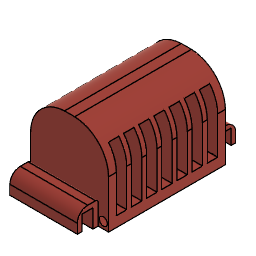
Tensor acoplable (Autodesk Fusion 360 design; units mm, degrees)
Autodesk Fusion 360 part; units mm, degrees
note: some values were not read from the file. Chosen so that the rebuilt part matches the saved one: which pieces of a blend or face edit are solid. Set by a fixed rule: which sketch regions a step uses.
sketch "Boceto1" plane through (0, 0, 0) normal (1, 0, 0) x (0, 1, 0)
  line L0 (0, 0) -> (0, 5)
  line L1 (0, 5) -> (4, 5)
  line L2 (4, 5) -> (4, 0)
  line L3 (4, 0) -> (53, 0)
  line L4 (53, 0) -> (53, 5)
  line L5 (53, 5) -> (57, 5)
  line L6 (57, 5) -> (57, 0)
  line L7 (-2, 0) -> (-2, 7)
  line L8 (-2, 7) -> (6, 7)
  line L9 (6, 7) -> (6, 2)
  line L10 (6, 2) -> (51, 2)
  line L11 (51, 2) -> (51, 7)
  line L12 (51, 7) -> (59, 7)
  line L13 (59, 7) -> (59, 0)
  line L14 (-2, 0) -> (0, 0)
  line L15 (59, 0) -> (57, 0)
  dimension "d1" = 5
  dimension "d2" = 4
  dimension "d3" = 49
  dimension "d4" = 5
  dimension "d5" = 4
  dimension "d6" = 5
  dimension "d7" = -2
  constraint coincident L0.start L14.end
  constraint vertical L0
  constraint perpendicular L0 L1
  constraint perpendicular L1 L2
  constraint perpendicular L2 L3
  constraint perpendicular L3 L4
  constraint perpendicular L4 L5
  constraint perpendicular L5 L6
  constraint perpendicular L0 L14
  constraint perpendicular L13 L15
  measures "d1" distance of L0.start L0.end
  measures "d2" distance of L0.end L1.end
  measures "d3" distance of L2.end L3.end
  measures "d4" distance of L3.end L4.end
  measures "d5" distance of L4.end L5.end
  measures "d6" distance of L5.end L6.end
extrude "Extruir1" add sketch "Boceto1" along normal blind 30 makes body 1
extrude "Extruir3" cut 1 faces at (10, 21, 2) along direction (0, 0, -1) blind 0.5 on bodies 1 bodies 1
sketch "Boceto2" plane through (0, 51, 0) normal (0, -1, 0) x (1, 0, 0)
  line L0 (0, 7) -> (0, 1.5)
  line L1 (30, 1.5) -> (30, 7)
  line L2 (30, 7) -> (0, 7)
  line L3 (0, 1.5) -> (30, 1.5)
  line L4 (15, 1.5) -> (15, 5)
  arc A0 (30, 1.5) -> (0, 1.5) centre (15, -28.8929) ccw
  dimension "d15" = 3.5
  constraint midpoint L3 L4.start
  constraint perpendicular L3 L4
  constraint coincident L4.end A0
  constraint coincident L1.start L3.end
  constraint coincident L0.end L3.start
  measures "d15" distance of L4.start L4.end
extrude "Extruir2" add sketch "Boceto2" along normal up to surface (45 mm away) contours L3 L4 A0 | L3 L4 A0 bodies 1
copy_body "Cuerpo - > Comp.1" bodies 1 removing the originals makes body 2 in component "Rodillo acoplable"
move_face "CarasDesfase1" offset -0.2 2 faces at (10, 57, 3.3333) (10, 0, 1.6667) on bodies 2 in component "Rodillo acoplable"
fillet "Empalme1" radius 4 2 edges at (15, -2, 7) (15, 59, 7) on bodies 2 in component "Rodillo acoplable"
fillet "Empalme2" radius 1 2 edges at (15, 6, 7) (15, 51, 7) on bodies 2 in component "Rodillo acoplable"
move_face "CarasDesfase2" offset 25 1 faces at (1.3409, 21, 2.1258) on bodies 2 in component "Rodillo acoplable"
fillet "Empalme3" radius 13.5 2 edges at (30, 28.5, 28.0577) (0, 28.5, 28.0577) on bodies 2 in component "Rodillo acoplable"
extrude "Extruir1'" add 2 faces at (10, -1.4, 0) (10, 58.4, 0) along direction (0, 0, -1) blind 1 on bodies 2 bodies 2 in component "Rodillo acoplable"
sketch "Boceto3" plane through (0, -0.2, 0) normal (0, 1, 0) x (-1, 0, 0)
  line L0 (0, -1) -> (0, 5)
  line L1 (0, 5) -> (-30, 5)
  line L2 (-30, 5) -> (-30, -1)
  line L3 (-30, -1) -> (0, -1)
  line L4 (0, -1) -> (-30, -1)
  line L5 (-30, -1) -> (-30, 1.5)
  line L6 (-30, 1.5) -> (0, 1.5)
  line L7 (0, 1.5) -> (0, -1)
  dimension "d38" = 2.5
  constraint horizontal L4
  constraint vertical L5
  constraint horizontal L6
  constraint vertical L7
  constraint coincident L2 L5.end
  constraint coincident L0.start L3.end
  measures "d38" distance of L2.end L5.end
extrude "Extruir9" add sketch "Boceto3" along normal blind 1.25 contours L0 L2 L3 L4 L5 L6 L7 bodies 2 in component "Rodillo acoplable"
sketch "Boceto4" plane through (0, 57.2, 0) normal (0, -1, 0) x (1, 0, 0)
  line L0 (0, 5) -> (0, -1)
  line L1 (0, -1) -> (30, -1)
  line L2 (30, -1) -> (30, 5)
  line L3 (30, 5) -> (0, 5)
  line L4 (0, -1) -> (30, -1)
  line L5 (30, -1) -> (30, 1.5)
  line L6 (30, 1.5) -> (0, 1.5)
  line L7 (0, 1.5) -> (0, -1)
  dimension "d27" = 2.5
  constraint horizontal L4
  constraint vertical L5
  constraint horizontal L6
  constraint vertical L7
  constraint coincident L0.end L1.start
  measures "d27" distance of L0.end L6.end
extrude "Extruir3'" add sketch "Boceto4" along normal blind 1.25 contours L0 L1 L2 L4 L5 L6 L7 bodies 2 in component "Rodillo acoplable"
extrude "Extruir4" add 1 faces at (20, 36.6667, 0) along direction (0, 0, -1) blind 1 on bodies 2 bodies 2 in component "Rodillo acoplable"
sketch "Boceto5" plane through (30, 0, 0) normal (1, 0, 0) x (0, 1, 0)
  line L0 (51, 16.4752) -> (6, 16.4752)
  line L1 (6, 16.4752) -> (6, 6)
  arc A0 (6, 6) -> (5, 7) centre (5, 6) ccw
  line L2 (5, 7) -> (2, 7)
  arc A1 (2, 7) -> (-2, 3) centre (2, 3) ccw
  line L3 (-2, 3) -> (-2, -1)
  line L4 (-2, -1) -> (-0.2, -1)
  line L5 (-0.2, 1.5) -> (-0.2, 5)
  line L6 (-0.2, 5) -> (4, 5)
  line L7 (4, 5) -> (4, -1)
  line L8 (4, -1) -> (53, -1)
  line L9 (53, -1) -> (53, 5)
  line L10 (53, 5) -> (57.2, 5)
  line L11 (57.2, 5) -> (57.2, 1.5)
  line L12 (57.2, 1.5) -> (55.95, 1.5)
  line L13 (55.95, 1.5) -> (55.95, -1)
  line L14 (55.95, -1) -> (59, -1)
  line L15 (59, -1) -> (59, 3)
  arc A2 (59, 3) -> (55, 7) centre (55, 3) ccw
  line L16 (55, 7) -> (52, 7)
  arc A3 (52, 7) -> (51, 6) centre (52, 6) ccw
  line L17 (51, 6) -> (51, 16.4752)
  line L18 (6, 6) -> (6, -1)
  line L19 (51, 6) -> (51, -1)
  line L20 (-0.2, -1) -> (-0.2, 1.5)
  constraint coincident L1.end A0.start
  constraint coincident L8 L18.end
  constraint tangent A0 L18
  constraint coincident A3.end L17.start
  constraint coincident L8 L19.end
  constraint tangent A3 L19
extrude "Extruir5" cut sketch "Boceto5" against normal blind 4 contours L8 L9 L10 L11 L12 L13 L14 L15 A2 L16 A3 L19 | A0 L2 A1 L3 L4 L5 L6 L7 L8 L18 L20 bodies 2 in component "Rodillo acoplable"
sketch "Boceto7" plane through (0, 51, 0) normal (0, 1, 0) x (-1, 0, 0)
  arc A0 (0, 16.4752) -> (-13.0539, 29.9678) centre (-13.5, 16.4752) ccw
  arc A1 (-13.0539, 29.9678) -> (-16.9461, 29.9678) centre (-15, -28.8929) ccw
  arc A2 (-16.9461, 29.9678) -> (-30, 16.4752) centre (-16.5, 16.4752) ccw
  line L0 (-30, 16.4752) -> (-30, -1)
  line L1 (-30, -1) -> (-26, -1)
  line L2 (-26, -1) -> (-26, 6)
  line L3 (-26, 6) -> (0, 6)
  line L4 (0, 6) -> (0, 16.4752)
  line L5 (-28, -1) -> (-28, 0.6)
  circle A3 centre (-28, 0.6) radius 1.55
  dimension "d41" = 1.6
  dimension "d42" = 3.1
  constraint midpoint L1 L5.start
  constraint perpendicular L1 L5
  constraint coincident L5.end A3.centre
  measures "d41" distance of L5.start L5.end
  measures "d42" diameter of A3
extrude "Extruir8" cut sketch "Boceto7" against normal blind 45 contours A3 bodies 2 in component "Rodillo acoplable"
extrude "Extruir10" cut 1 faces at (30, 0.2167, -0.1667) along direction (-1, 0, 0) up to surface (4 mm away) on bodies 2 bodies 2 in component "Rodillo acoplable"
extrude "Extruir11" add sketch "Boceto7" against normal blind 42 contours A3 bodies 2 in component "Rodillo acoplable"
extrude "Extruir12" cut sketch "Boceto7" against normal blind 3 contours A3 bodies 2 in component "Rodillo acoplable"
extrude "Extruir13" cut 2 faces at (17.3333, 2.6, 5) (8.6667, 54.4, 5) along direction (0, 0, 1) blind 0.15 on bodies 2 bodies 2 in component "Rodillo acoplable"
sketch "Boceto8" plane through (30, 0, 0) normal (1, 0, 0) x (0, 1, 0)
  line L0 (6, 16.4752) -> (6, -1)
  line L1 (6, -1) -> (51, -1)
  line L2 (51, -1) -> (51, 16.4752)
  line L3 (51, 16.4752) -> (6, 16.4752)
  line L4 (6, -1) -> (9, -1)
  line L5 (9, -1) -> (9, 2)
  line L6 (9, 2) -> (13, 2)
  line L7 (13, 2) -> (13, 25)
  line L8 (13, 25) -> (9, 25)
  line L9 (9, 25) -> (9, 2)
  line L10 (18.8333, 2) -> (18.8333, 25)
  line L11 (18.8333, 25) -> (14.8333, 25)
  line L12 (14.8333, 25) -> (14.8333, 2)
  line L13 (14.8333, 2) -> (18.8333, 2)
  line L14 (24.6667, 2) -> (24.6667, 25)
  line L15 (24.6667, 25) -> (20.6667, 25)
  line L16 (20.6667, 25) -> (20.6667, 2)
  line L17 (20.6667, 2) -> (24.6667, 2)
  line L18 (30.5, 2) -> (30.5, 25)
  line L19 (30.5, 25) -> (26.5, 25)
  line L20 (26.5, 25) -> (26.5, 2)
  line L21 (26.5, 2) -> (30.5, 2)
  line L22 (36.3333, 2) -> (36.3333, 25)
  line L23 (36.3333, 25) -> (32.3333, 25)
  line L24 (32.3333, 25) -> (32.3333, 2)
  line L25 (32.3333, 2) -> (36.3333, 2)
  line L26 (42.1667, 2) -> (42.1667, 25)
  line L27 (42.1667, 25) -> (38.1667, 25)
  line L28 (38.1667, 25) -> (38.1667, 2)
  line L29 (38.1667, 2) -> (42.1667, 2)
  line L30 (48, 2) -> (48, 25)
  line L31 (48, 25) -> (44, 25)
  line L32 (44, 25) -> (44, 2)
  line L33 (44, 2) -> (48, 2)
  dimension "d55" = 4
  dimension "d56" = 23
  dimension "d59" = 35
  dimension "d60" = 0
  constraint coincident L0.end L1.start
  constraint coincident L1 L4.end
  constraint perpendicular L4 L5
  constraint horizontal L6
  constraint vertical L7
  constraint horizontal L8
  constraint vertical L9
  measures "d55" distance of L5.end L6.end
  measures "d56" distance of L5.end L8.end
extrude "Extruir14" cut sketch "Boceto8" against normal blind 37 contours L3 L7 L8 L9 | L3 L6 L7 L9 | L3 L10 L11 L12 | L3 L10 L12 L13 | L3 L30 L32 L33 | L3 L30 L31 L32 | L3 L14 L15 L16 | L3 L14 L16 L17 | L3 L26 L28 L29 | L3 L26 L27 L28 | L3 L18 L19 L20 | L3 L18 L20 L21 | L3 L22 L24 L25 | L3 L22 L23 L24 bodies 2 in component "Rodillo acoplable"
extrude "Extruir15" add 1 faces at (8.6667, 21, -1) along direction (0, 0, -1) blind 1 on bodies 2 bodies 2 in component "Rodillo acoplable"
extrude "Extruir16" add 2 faces at (17.3333, 0.6333, 1.5) (17.3333, 56.7833, 1.5) along direction (0, 0, 1) blind 0.4 on bodies 2 bodies 2 in component "Rodillo acoplable"
extrude "Extruir18" cut 2 faces at (8.6667, -0.3833, -1) (8.6667, 57.9833, -1) along direction (0, 0, 1) blind 0.3 on bodies 2 bodies 2 in component "Rodillo acoplable"
extrude "Extruir19" cut 2 faces at (17.3333, 0.6333, 1.9) (17.3333, 56.7833, 1.9) along direction (0, 0, -1) blind 7 on bodies 2 bodies 2 in component "Rodillo acoplable"
component "Rodillo acoplable" placed x (1, 0, 0) y (0, 1, 0) z (0, 0, 1) at (0, 0, 0)
named bodies: "Rodillo acoplable"
